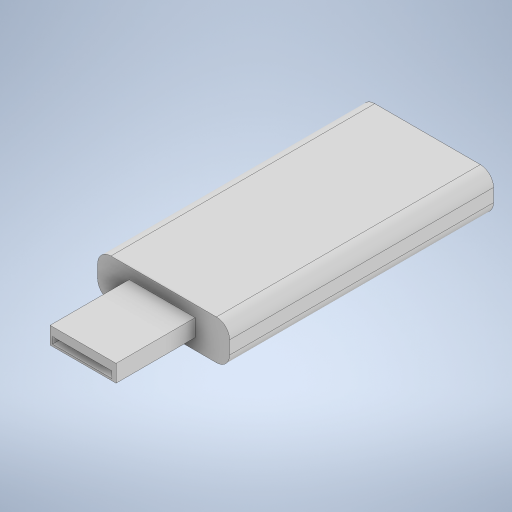
# Autodesk Inventor part: USB
Saved by Autodesk Inventor 2024.2 (Build 282272000, 272)
## iProperties
Created: 2024-02-29
Part Number: USB
Material: 一般
Document SubType Name: Modeling
Designer: User
Density: 1 g/cm^3
Appearance: 預設
Mass: 0.608332 g
Surface Area: 6.79547 cm^2
Volume: 0.608332 cm^3
Author: User
Autodesk Inventor part; units mm, degrees
ref_plane "YZ Plane" through (0, 0, 0) normal (1, 0, 0) x (0, 1, 0)
ref_plane "XZ Plane" through (0, 0, 0) normal (0, 1, 0) x (-1, 0, 0)
ref_plane "XY Plane" through (0, 0, 0) normal (0, 0, 1) x (1, 0, 0)
sketch "草圖2" plane through (0, 0, 0) normal (0, 1, 0) x (-1, 0, 0)
  line L0 (0, 0) -> (10, 0)
  line L1 (10, 0) -> (10, -20)
  line L2 (10, -20) -> (0, -20)
  line L3 (0, -20) -> (0, 0)
  dimension "d1" = 10
  dimension "d2" = 20
  constraints: 8 end point, 2 parallel, 1 horizontal, 1 perpendicular
  measures "d1" distance of L1.end L2.end
  measures "d2" distance of L0.end L1.end
extrude "擠出1" add sketch "草圖2" along normal blind 3
fillet "圓角1" radius 1 4 edges at (-10, 3, -10) (0, 3, -10) (0, 0, -10) (-10, 0, -10)
sketch "草圖3" plane through (-9, 0, 0) normal (0, 0, 1) x (1, 0, 0)
  line L0 (1.3959, 0.8511) -> (6.3959, 0.8511)
  line L1 (6.3959, 0.8511) -> (6.3959, 2.1511)
  line L2 (6.3959, 2.1511) -> (1.3959, 2.1511)
  line L3 (1.3959, 2.1511) -> (1.3959, 0.8511)
  point P0 (9, 0)
  dimension "d6" = 5
  dimension "d7" = 1.3
  constraints: 8 end point, 2 parallel, 1 horizontal, 1 perpendicular
  measures "d6" distance of L2.end L1.end
  measures "d7" distance of L1.end L0.end
extrude "擠出2" add sketch "草圖3" along normal blind 6
sketch "草圖4" plane through (-9, 0, 6) normal (0, 0, 1) x (1, 0, 0)
  line L0 (6.0686, 1.499) -> (1.5686, 1.499)
  line L1 (1.5686, 1.499) -> (1.5686, 0.999)
  line L2 (1.5686, 0.999) -> (6.0686, 0.999)
  line L3 (6.0686, 0.999) -> (6.0686, 1.499)
  line L4 (4.9801, 1.499) -> (4.9403, 1.499)
  point P0 (9, 0)
  dimension "d12" = 4.5
  dimension "d13" = 0.5
  constraints: 10 end point, 2 horizontal, 2 parallel, 1 perpendicular, 1 point on line
  measures "d12" distance of L0.start L0.end
  measures "d13" distance of L2.end L0.start
extrude "擠出3" cut sketch "草圖4" against normal blind 6
